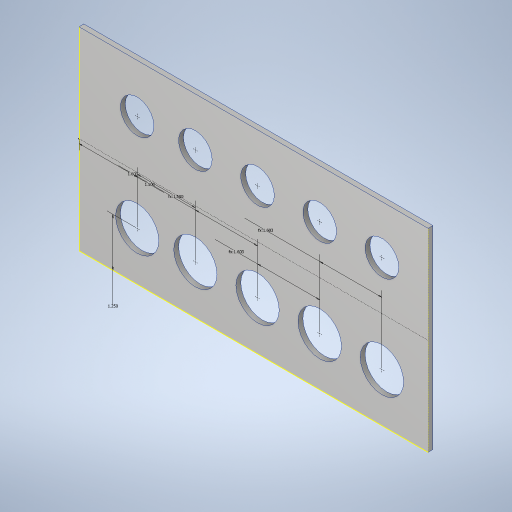
# Autodesk Inventor part: BEARING TEST
Saved by Autodesk Inventor 2023.4 (Build 274418000, 418)
## iProperties
Created: 2025-01-19
Part Number: BEARING TEST
Material: Aluminum 6061
Document SubType Name: Modeling
Designer: jmcintyr
Density: 2.7 g/cm^3
Appearance: Aluminum - Flat
Author: jmcintyr
Autodesk Inventor part; units mm, degrees
ref_plane "YZ Plane" through (0, 0, 0) normal (1, 0, 0) x (0, 1, 0)
ref_plane "XZ Plane" through (0, 0, 0) normal (0, 1, 0) x (-1, 0, 0)
ref_plane "XY Plane" through (0, 0, 0) normal (0, 0, 1) x (1, 0, 0)
sketch "Sketch1" plane through (0, 0, 0) normal (0, 0, 1) x (1, 0, 0)
  line L0 (0, 0) -> (228.6, 0)
  line L1 (228.6, 0) -> (228.6, 127)
  line L2 (228.6, 127) -> (0, 127)
  line L3 (0, 127) -> (0, 0)
  dimension "d0" = 228.6
  dimension "d1" = 127
  constraints: 8 end point, 2 parallel, 1 horizontal, 1 perpendicular
  measures "d0" distance of L2.end L1.end
  measures "d1" distance of L1.end L0.end
extrude "Extrusion1" add sketch "Sketch1" against normal blind 3.175
sketch "Sketch2" plane through (0, 0, 0) normal (0, 0, 1) x (1, 0, 0)
  line L0 (0, 0) -> (228.6, 0) projected
  line L1 (0, 127) -> (0, 0) projected
  point P0 (38.1, 31.75)
  point P1 (76.2, 31.75)
  point P2 (116.9154, 31.75)
  point P3 (157.6309, 31.75)
  point P4 (198.3463, 31.75)
  point P5 (0, 63.5)
  dimension "d4" = 31.75
  dimension "d5" = 38.1
  dimension "d6" = 38.1
  dimension "d7" = 40.7154
  dimension "d8" = 40.7154
  dimension "d9" = 40.7154
  constraints: 4 horizontal alignment, 1 midpoint
  measures "d4" distance from line of L0 point (38.1, 31.75)
  measures "d5" horizontal distance of point (0, 63.5) point (38.1, 31.75)
  measures "d6" distance of point (76.2, 31.75) point (38.1, 31.75)
  measures "d7" distance of point (76.2, 31.75) point (116.915, 31.75)
  measures "d8" distance of point (116.915, 31.75) point (157.631, 31.75)
  measures "d9" distance of point (157.631, 31.75) point (198.346, 31.75)
hole "Hole1" at (38.1, 31.75, 0) direction (0, 0, -1) diameter 28.2956 end through all
hole "Hole2" at (76.2, 31.75, 0) direction (0, 0, -1) diameter 28.321 end through all
hole "Hole3" at (116.9154, 31.75, 0) direction (0, 0, -1) diameter 28.3464 end through all
hole "Hole4" at (157.6309, 31.75, 0) direction (0, 0, -1) diameter 28.4734 end through all
hole "Hole5" at (198.3463, 31.75, 0) direction (0, 0, -1) diameter 28.3972 end through all
sketch "Sketch3" plane through (0, 0, 0) normal (0, 0, 1) x (1, 0, 0)
  line L0 (0, 0) -> (0, 127) construction
  line L1 (0, 63.5) -> (228.6, 63.5) construction
  line L2 (228.6, 127) -> (228.6, 0) construction
  point P0 (38.1, 31.75)
  point P1 (76.2, 31.75)
  point P2 (116.9154, 31.75)
  point P3 (157.6309, 31.75)
  point P4 (198.3463, 31.75)
  point P5 (38.1, 95.25)
  point P6 (76.2, 95.25)
  point P7 (116.9154, 95.25)
  point P8 (157.6309, 95.25)
  point P9 (198.3463, 95.25)
  constraints: 5 symmetric about line, 2 end point, 2 midpoint
hole "Hole6" at (38.1, 95.25, 0) direction (0, 0, -1) diameter 21.971 end through all
hole "Hole7" at (76.2, 95.25, 0) direction (0, 0, -1) diameter 21.971 end through all
hole "Hole8" at (116.9154, 95.25, 0) direction (0, 0, -1) diameter 21.9964 end through all
hole "Hole9" at (157.6309, 95.25, 0) direction (0, 0, -1) diameter 22.0218 end through all
hole "Hole10" at (198.3463, 95.25, 0) direction (0, 0, -1) diameter 22.0472 end through all
equation "\"d6\" = d5"
equation "\"d8\" = d7"
equation "\"d9\" = d7"
body "Solid1"
